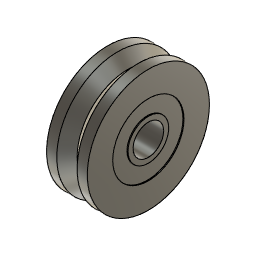
Omni_wheel_r18 v1 (Autodesk Fusion 360 archive; units mm, degrees)
design "rollers"
Autodesk Fusion 360 part; units mm, degrees
sketch "Sketch2" plane through (0, 0, 0) normal (0, 0, 1) x (1, 0, 0)
  line L0 (0, 0) -> (0, 6)
  line L1 (4, 6) -> (4, 0)
  line L2 (4, 0) -> (0, 0)
  line L3 (1, 6) -> (2, 5)
  line L4 (2, 5) -> (3, 6)
  line L5 (0, 6) -> (1, 6)
  line L6 (3, 6) -> (4, 6)
  dimension "d12" = 4
  dimension "d13" = 1
  dimension "d14" = 1
  dimension "d15" = 6
  constraint coincident L0.start L2.end
  constraint coincident L4.end L5
  constraint perpendicular L3 L4
  constraint perpendicular L0 L2
  constraint vertical L0
  constraint horizontal L6
  measures "d12" distance of L0 L1
  measures "d13" distance of L0.end L3.start
  measures "d14" distance of L1.start L4.end
  measures "d15" distance of L2 L5
revolve "Revolve1" add sketch "Sketch2" angle 360 about axis through (4, 0, 0) along (-1, 0, 0)
sketch "Sketch3" plane through (4, 0, 0) normal (1, 0, 0) x (0, 1, 0)
  circle A0 centre (0, 0) radius 6
  circle A1 centre (0, 0) radius 1.5
  dimension "d18" = 3
  constraint coincident A0.centre A1.centre
  measures "d18" diameter of A1
extrude "Extrude2" cut sketch "Sketch3" against normal through all contours A1
sketch "Sketch4" plane through (4, 0, 0) normal (1, 0, 0) x (0, 1, 0)
  circle A0 centre (0, 0) radius 1.5
  circle A1 centre (0, 0) radius 6
  circle A2 centre (0, 0) radius 3.5
  circle A3 centre (0, 0) radius 2
  dimension "d20" = 7
  dimension "d21" = 4
  constraint coincident A0.centre A1.centre
  constraint concentric A2 A3
  measures "d20" diameter of A2
  measures "d21" diameter of A3
extrude "Extrude3" cut sketch "Sketch4" against normal blind 0.1 contours A2
sketch "Sketch5" plane through (0, 0, 0) normal (-1, 0, 0) x (0, -1, 0)
  circle A0 centre (0, 0) radius 1.5
  circle A1 centre (0, 0) radius 6
  circle A2 centre (0, 0) radius 2
  circle A3 centre (0, 0) radius 3.5
  dimension "d24" = 7
  dimension "d25" = 4
  constraint coincident A0.centre A1.centre
  measures "d24" diameter of A3
  measures "d25" diameter of A2
extrude "Extrude4" cut sketch "Sketch5" against normal blind 0.1 contours A3
